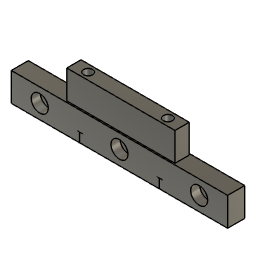
General Purpose Mounting Block B v19 (Autodesk Fusion 360 design; units mm, degrees)
Autodesk Fusion 360 part; units mm, degrees
sketch "Schizzo7" plane through (0, 0, 0) normal (0, 0, 1) x (1, 0, 0)
  line L0 (-81.9529, 9.2169) -> (-5.9529, 9.2169)
  line L1 (-5.9529, 9.2169) -> (-5.9529, 3.2169)
  line L2 (-5.9529, 3.2169) -> (-81.9529, 3.2169)
  line L3 (-81.9529, 3.2169) -> (-81.9529, 9.2169)
  line L4 (-81.9529, 6.2169) -> (-5.9529, 6.2169) construction
  line L5 (-43.9529, 9.2169) -> (-43.9529, 3.2169) construction
  line L6 (-6.4657, 3.7169) -> (-81.4401, 3.7169)
  line L7 (-81.4401, 3.7169) -> (-81.4401, 8.7169)
  line L8 (-81.4401, 8.7169) -> (-6.4657, 8.7169)
  line L9 (-6.4657, 8.7169) -> (-6.4657, 3.7169)
  line L10 (-6.4657, 3.7169) -> (-81.4401, 8.7169) construction
  line L11 (-81.4401, 3.7169) -> (-6.4657, 8.7169) construction
  circle A0 centre (-57.9529, 6.2169) radius 3
  circle A1 centre (-57.9529, 6.2169) radius 1.6
  circle A2 centre (-29.9529, 6.2169) radius 1.6
  circle A3 centre (-29.9529, 6.2169) radius 3
  line L12 (-49.5331, 8.6997) -> (-38.3727, 8.734) construction
  line L13 (-38.3727, 8.734) -> (-38.3574, 3.7461) construction
  line L14 (-38.3574, 3.7461) -> (-49.5178, 3.7118) construction
  line L15 (-49.5178, 3.7118) -> (-49.5331, 8.6997) construction
  line L16 (-62.9529, 3.7169) -> (-62.9529, 8.7169)
  line L17 (-24.9529, 3.7169) -> (-24.9529, 8.7169)
  point P0 (-43.9529, 6.2169)
  dimension "d44" = 76
  dimension "d45" = 6
  dimension "d46" = 5
  dimension "d47" = 6
  dimension "d48" = 3.2
  dimension "d49" = 28
  dimension "d60" = 5
  dimension "d72" = 38
  text T0 "28" font "Arial" height 5 bold align left top in box 11.1605 x 4.988 at (-49.5331, 8.6997) x (0.999995, 0.00307) y (0.00307, -0.999995) spacing 1 kerned
  constraint horizontal L0
  constraint vertical L1
  constraint horizontal L2
  constraint vertical L3
  constraint midpoint L3 L4.start
  constraint midpoint L1 L4.end
  constraint midpoint L0 L5.start
  constraint midpoint L2 L5.end
  constraint horizontal L6
  constraint perpendicular L6 L7
  constraint parallel L6 L8
  constraint parallel L7 L9
  constraint coincident L10 P0
  constraint coincident L11 P0
  constraint midpoint L5 P0
  constraint coincident L4 A0.centre
  constraint concentric A0 A1
  constraint symmetric L5 A0 A3
  constraint symmetric L5 A1 A2
  constraint midpoint L8
  constraint coincident L6 L16.start
  constraint coincident L8 L16.end
  constraint perpendicular L8 L16
  constraint symmetric L5 L16.start L17.start
  constraint symmetric L5 L16.end L17.end
  measures "d44" distance of L0.start L0.end
  measures "d45" distance of L0.start L2.end
  measures "d46" distance of L6.end L7.end
  measures "d47" diameter of A0
  measures "d48" diameter of A1
  measures "d49" distance of A0.centre A2.centre
  measures "d72" distance of L16 L17
extrude "Estrusione11" add sketch "Schizzo7" along normal blind 10
extrude "Estrusione12" add sketch "Schizzo7" along normal blind 20 contours L6 L8 A0 | L6 L8 A0 A3 | L6 L8 A0 L16 | L6 L8 A3 | L6 L8 A3 L17
extrude "Estrusione13" cut sketch "Schizzo7" along normal blind 3.2 contours L8 A0 | L8 A3 | L6 L8 A0 | L6 A0 | L6 L8 A3 | L6 A3
extrude "Estrusione17" cut sketch "Schizzo7" along normal blind 1 text T0
sketch "Schizzo9" plane through (0, 3.2169, 0) normal (0, -1, 0) x (1, 0, 0)
  line L0 (-29.9529, 0) -> (-5.9529, 0)
  line L1 (-5.9529, 0) -> (-5.9529, 10)
  line L2 (-5.9529, 10) -> (-81.9529, 10)
  line L3 (-81.9529, 10) -> (-81.9529, 0)
  line L4 (-81.9529, 10) -> (-5.9529, 10) construction
  line L5 (-5.9529, 10) -> (-5.9529, 0) construction
  line L6 (-5.9529, 0) -> (-81.9529, 0) construction
  line L7 (-81.9529, 0) -> (-81.9529, 10) construction
  line L8 (-81.9529, 5) -> (-5.9529, 5) construction
  circle A0 centre (-15.9529, 5) radius 1.6
  circle A1 centre (-15.9529, 5) radius 3
  circle A2 centre (-71.9529, 5) radius 1.6
  circle A3 centre (-71.9529, 5) radius 3
  circle A4 centre (-43.9529, 5) radius 3
  circle A5 centre (-43.9529, 5) radius 1.6
  line L9 (-81.9529, 0) -> (-57.9529, 0)
  line L10 (-57.9529, 0) -> (-29.9529, 0)
  line L11 (-43.9529, 0) -> (-43.9529, 10) construction
  dimension "d63" = 3.2
  dimension "d64" = 6
  dimension "d65" = 3.2
  dimension "d66" = 6
  dimension "d75" = 76
  dimension "d76" = 28
  dimension "d77" = 28
  constraint horizontal L4
  constraint vertical L5
  constraint horizontal L6
  constraint vertical L7
  constraint coincident L0.end L1.start
  constraint coincident L2.end L3.start
  constraint midpoint L7 L8.start
  constraint midpoint L5 L8.end
  constraint concentric A0 A1
  constraint coincident L8 A2.centre
  constraint concentric A2 A3
  constraint coincident L8 A4.centre
  constraint coincident A4.centre A5.centre
  constraint midpoint L10 L11.start
  constraint midpoint L4 L11.end
  constraint coincident A4.centre L11
  measures "d63" diameter of A0
  measures "d64" diameter of A1
  measures "d65" diameter of A2
  measures "d66" diameter of A3
  measures "d75" distance of L5 L7
  measures "d76" distance of A2.centre A4.centre
  measures "d77" distance of A0.centre A4.centre
extrude "Estrusione15" cut sketch "Schizzo9" against normal blind 10 contours A0 | A2 | A5
extrude "Estrusione16" cut sketch "Schizzo9" against normal blind 3.2 contours A1 | A3 | A4
equation "d65 = d63"
equation "d66 = d64"
named bodies: "Block-20-10 to 5"
